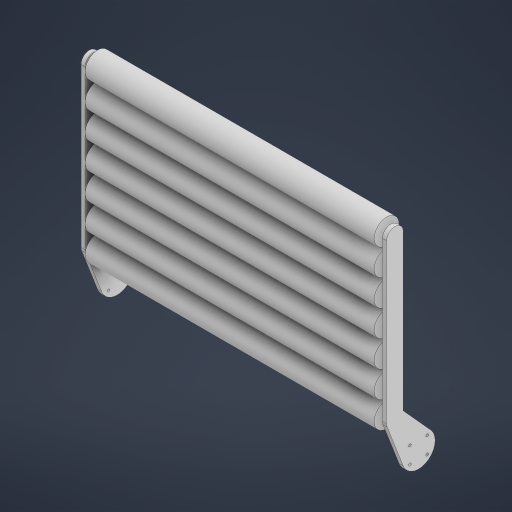
# Autodesk Inventor part: Orienter
Saved by Autodesk Inventor 2023 (Build 270158000, 158)
## iProperties
Created: 2023-11-05
Part Number: Orienter
Material: Generic
Document SubType Name: Modeling
Designer: Abhinav
Density: 1 g/cm^3
Appearance: Default
Author: Abhinav
Autodesk Inventor part; units mm, degrees
ref_plane "YZ Plane" through (0, 0, 0) normal (1, 0, 0) x (0, 1, 0)
ref_plane "XZ Plane" through (0, 0, 0) normal (0, 1, 0) x (-1, 0, 0)
ref_plane "XY Plane" through (0, 0, 0) normal (0, 0, 1) x (1, 0, 0)
sketch "Sketch1" plane through (0, 0, 0) normal (1, 0, 0) x (0, 1, 0)
  line L0 (-0.1455, -0.2526) -> (28.1388, 28.0317)
  line L1 (-0.1455, -0.2526) -> (39.8545, -0.2526) construction
  arc A0 (-7.3244, 18.4146) -> (13.2595, -15.0953) centre (-0.1455, -0.2526) ccw
  line L2 (26.5, 28.4) -> (87.1548, 28.4)
  line L3 (26.5, 28.4) -> (46.5, 28.4) construction
  circle A1 centre (46.5, 28.4) radius 15 construction
  circle A2 centre (78.5, 28.4) radius 15 construction
  circle A3 centre (110.5, 28.4) radius 15 construction
  circle A4 centre (142.5, 28.4) radius 15 construction
  circle A5 centre (174.5, 28.4) radius 15 construction
  line L4 (174.5, 28.4) -> (46.5, 28.4) construction
  line L5 (174.5, 38.4) -> (46.5, 38.4)
  line L6 (50.3473, 18.4) -> (174.5, 18.4)
  arc A6 (46.5, 38.4) -> (46.5, 18.4) centre (46.5, 28.4) ccw construction
  line L7 (13.2595, -15.0953) -> (50.3473, 18.4)
  line L8 (-7.3244, 18.4146) -> (42.9106, 37.7336)
  arc A7 (46.5, 18.4) -> (53.2025, 20.9786) centre (46.5, 28.4) ccw construction
  arc A8 (46.5, 38.4) -> (42.9106, 37.7336) centre (46.5, 28.4) ccw
  circle A9 centre (46.5, 28.4) radius 2.5
  circle A10 centre (78.5, 28.4) radius 2.5
  circle A11 centre (110.5, 28.4) radius 2.5
  circle A12 centre (142.5, 28.4) radius 2.5
  circle A13 centre (174.5, 28.4) radius 2.5
  circle A14 centre (206.5, 28.4) radius 2.5
  circle A15 centre (238.5, 28.4) radius 2.5
  circle A16 centre (206.5, 28.4) radius 15 construction
  circle A17 centre (238.5, 28.4) radius 15 construction
  line L9 (174.5, 28.4) -> (238.5, 28.4) construction
  line L10 (174.5, 38.4) -> (238.5, 38.4)
  line L11 (238.5, 18.4) -> (174.5, 18.4)
  arc A18 (238.5, 18.4) -> (238.5, 38.4) centre (238.5, 28.4) ccw
  line L12 (-0.1455, -0.2526) -> (-10.1789, -10.7207) construction
  line L13 (-0.1455, -0.2526) -> (9.8879, -10.7207) construction
  line L14 (-0.1455, -0.2526) -> (-10.1789, 10.2155) construction
  line L15 (-0.1455, -0.2526) -> (9.8879, 10.2155) construction
  circle A19 centre (-10.1789, -10.7207) radius 1.5
  circle A20 centre (9.8879, -10.7207) radius 1.5
  circle A21 centre (-10.1789, 10.2155) radius 1.5
  circle A22 centre (9.8879, 10.2155) radius 1.5
  point P0 (0, 0)
  point P1 (110.5, 28.4)
  dimension "d4" = 40
  dimension "d5" = 45
  dimension "d9" = 20
  dimension "d10" = 32
  dimension "d11" = 20
  dimension "d13" = 5
  dimension "d16" = 32
  dimension "d38" = 20
  dimension "d39" = 14.5
  dimension "d40" = 14.5
  dimension "d41" = 3
  constraints: 36 end point, 23 centre point, 10 point on circle, 8 coincident, 8 tangent, 5 horizontal, 3 equal radius, 2 midpoint, 2 parallel, 2 point on line, 2 symmetric about line, 1 collinear, 1 equal length, 26 other
  measures "d4" distance of L0.start L0.end
  measures "d5" angle of L1 L0
  measures "d9" distance of L2.start L3.end
  measures "d10" distance of L4.end A2.centre
  measures "d11" diameter of A6
  measures "d13" diameter of A9
  measures "d16" distance of A9.centre A10.centre
  measures "d38" radius of A0
  measures "d39" distance of L12.start L12.end
  measures "d40" distance of L12.start L13.end
  measures "d41" diameter of A19
extrude "Extrusion1" add sketch "Sketch1" along normal blind 5 contours L8 A8 L5 L10 A18 L11 L6 L7 A0 | A9 L2 | L2 A9 | A10 L2 | L2 A10 | A11 | A12 | A13 | A14 | A15
sketch "Sketch2" plane through (5, 0, 0) normal (1, 0, 0) x (0, 0, -1)
  circle A0 centre (-28.4, 46.5) radius 2.5 projected
  circle A1 centre (-28.4, 238.5) radius 2.5 projected
  circle A2 centre (-28.4, 46.5) radius 2.5 projected
  circle A3 centre (-28.4, 238.5) radius 2.5 projected
  line L0 (-28.4, 46.5) -> (-28.4, 238.5) construction
  line L1 (-13.4, 46.5) -> (-13.4, 238.5)
  line L2 (-43.4, 238.5) -> (-43.4, 46.5)
  arc A4 (-43.4, 46.5) -> (-13.4, 46.5) centre (-28.4, 46.5) ccw
  arc A5 (-13.4, 238.5) -> (-43.4, 238.5) centre (-28.4, 238.5) ccw
  circle A6 centre (-28.4, 206.5) radius 2.5 projected
  circle A7 centre (-28.4, 174.5) radius 2.5 projected
  circle A8 centre (-28.4, 142.5) radius 2.5 projected
  circle A9 centre (-28.4, 110.5) radius 2.5 projected
  circle A10 centre (-28.4, 78.5) radius 2.5 projected
  point P0 (0, 0)
  dimension "d27" = 30
  constraints: 8 end point, 4 point on circle, 4 tangent, 2 centre point, 1 midpoint, 1 parallel
  measures "d27" diameter of A5
extrude "Extrusion2" add sketch "Sketch2" along normal blind 5 contours A0 | A1 | A6 | A7 | A8 | A9 | A10
sketch "Sketch3" plane through (10, 238.5, 28.4) normal (1, 0, 0) x (0, 0, -1)
  circle A0 centre (0, 0) radius 2.5 projected
  circle A1 centre (0, 0) radius 15
  line L0 (0, 0) -> (0, -15) construction
  circle A2 centre (0, -32) radius 15
  circle A3 centre (0, -64) radius 15
  circle A4 centre (0, -96) radius 15
  circle A5 centre (0, -128) radius 15
  circle A6 centre (0, -160) radius 15
  circle A7 centre (0, -192) radius 15
  point P0 (28.4, -238.5)
  point P1 (0, -47)
  point P2 (0, -79)
  point P3 (0, -111)
  point P4 (0, -143)
  point P5 (0, -175)
  point P6 (0, -207)
  dimension "d28" = 30
  dimension "d31" = 32
  constraints: 7 vertical, 7 vertical alignment, 2 end point, 1 coincident, 26 other
  measures "d31" distance of L0.start point (0, -32)
extrude "Extrusion3" add sketch "Sketch3" along normal blind 175 contours A0 | A1 | A2 | A3 | A4 | A5 | A6 | A7
ref_plane "Work Plane1" through (185, 0, 0) normal (1, 0, 0) x (0, 0, -1)
mirror "Mirror2" about plane through (185, 0, 0) normal (1, 0, 0) of "Extrusion1", "Extrusion2", "Extrusion3"
body "Solid1"
